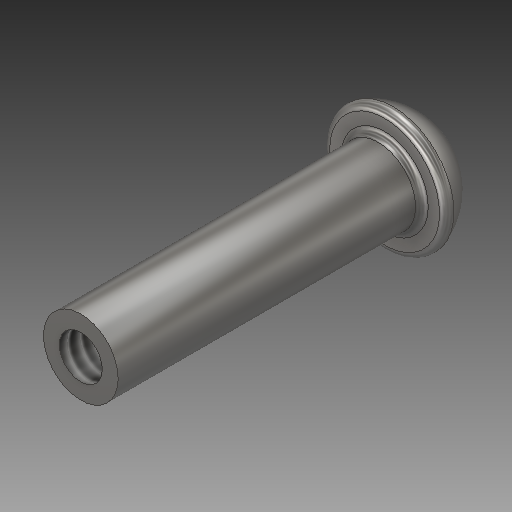
# Autodesk Inventor part: Part3
Saved by Autodesk Inventor 2018 (Build 220112000, 112)
## iProperties
Created: 2018-04-06
Part Number: Part3
Material: Stainless Steel
Document SubType Name: Modeling
Designer: 232963
Density: 8 g/cm^3
Appearance: Semi-Polished
Mass: 1.51811 g
Surface Area: 3.04468 cm^2
Volume: 0.189764 cm^3
Author: 232963
Autodesk Inventor part; units mm, degrees
ref_plane "YZ Plane" through (0, 0, 0) normal (1, 0, 0) x (0, 1, 0)
ref_plane "XZ Plane" through (0, 0, 0) normal (0, 1, 0) x (-1, 0, 0)
sketch "Sketch1" plane through (0, 0, 0) normal (0, 0, 1) x (1, 0, 0)
  circle A0 centre (0, 0) radius 1.8733
  dimension "d0" = 3.7465
  constraints: 1 centre point, 1 coincident
  measures "d0" diameter of A0
extrude "Extrusion1" add sketch "Sketch1" along normal blind 15.24
sketch "Sketch2" plane through (0, 0, 0) normal (0, 0, -1) x (-1, 0, 0)
  circle A0 centre (0, 0) radius 1.8732 projected
  circle A1 centre (0, 0) radius 3.175
  dimension "d3" = 6.35
  constraints: 1 centre point, 1 coincident
  measures "d3" diameter of A1
extrude "Extrusion2" add sketch "Sketch2" along normal blind 2.54 contours A0 | A1
fillet "Fillet1" radius 3.175 1 edges at (3.175, 0, -2.54)
fillet "Fillet2" radius 0.3175 1 edges at (3.175, 0, 0)
fillet "Fillet3" radius 0.3175 1 edges at (-1.8733, 0, 0)
ref_plane "Work Plane1" through (0, 0, -5.3975) normal (0, 0, 1) x (1, 0, 0)
sketch "Sketch4" plane through (0, 0, -5.3975) normal (0, 0, 1) x (1, 0, 0)
  line L0 (1.3748, 0) -> (0.6874, -1.1906)
  line L1 (0.6874, -1.1906) -> (-0.6874, -1.1906)
  line L2 (-0.6874, -1.1906) -> (-1.3748, 0)
  line L3 (-1.3748, 0) -> (-0.6874, 1.1906)
  line L4 (-0.6874, 1.1906) -> (0.6874, 1.1906)
  line L5 (0.6874, 1.1906) -> (1.3748, 0)
  point P0 (0, 0)
  point P1 (0, 0)
  dimension "d19" = 2.3813
  constraints: 12 end point, 1 coincident, 13 other
  measures "d19" distance between parallel lines of L1 L4
extrude "Extrusion3" cut sketch "Sketch4" along normal blind 4.1275
sketch "Sketch5" plane through (0, 0, 15.24) normal (0, 0, 1) x (1, 0, 0)
  point P0 (0, 0)
hole "Hole1" at (0, 0, 15.24) direction (0, 0, -1) diameter 2.159 depth 5.6896 tip angle 118
body "Solid1"
